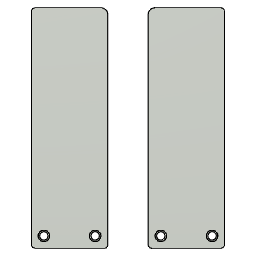
mriya-cnc-mcu-cover-v1.01 (Autodesk Fusion 360 design; units mm, degrees)
Autodesk Fusion 360 part; units mm, degrees
sketch "mriya-mcu-cover" plane through (0, 0, 0) normal (0, 0, 1) x (1, 0, 0)
  line L0 (-22.7, 5) -> (-5.8, 5) construction
  line L1 (-5, 5.8) -> (-5, 62) construction
  arc A0 (-5.8, 5) -> (-5, 5.8) centre (-5.8, 5.8) ccw construction
  arc A1 (-23.5, 5.8) -> (-22.7, 5) centre (-22.7, 5.8) ccw construction
  line L2 (-4.9, 5) -> (-4.9, 62)
  line L3 (-23.5, 5.8) -> (-23.5, 62.7) construction
  line L4 (-23.5, 63.6) -> (-6.5, 63.6)
  arc A2 (-10, 62.8) -> (-9.3, 63.5) centre (-10, 63.5) ccw construction
  arc A3 (-19.3, 63.5) -> (-18.6, 62.8) centre (-18.6, 63.5) ccw construction
  line L5 (-18.6, 62.8) -> (-10, 62.8) construction
  arc A4 (-22.7, 63.5) -> (-23.5, 62.7) centre (-22.7, 62.7) ccw construction
  line L6 (-22.7, 63.5) -> (-6.5, 63.5) construction
  line L7 (-23.5, 5) -> (-4.9, 5)
  circle A5 centre (-8, 8) radius 1.4
  circle A6 centre (-20.5, 8) radius 1.4
  line L8 (-23.5, 5) -> (-23.5, 63.6)
  arc A7 (-5, 62) -> (-6.5, 63.5) centre (-6.5, 62) ccw construction
  arc A8 (-4.9, 62) -> (-6.5, 63.6) centre (-6.5, 62) ccw
  circle A9 centre (-20.5, 8) radius 1
  circle A10 centre (-8, 8) radius 1
  line L9 (-5, 23.7) -> (-4.9, 23.7)
  dimension "d601" = 2.8
  dimension "d602" = 2.8
  dimension "d609" = 2
  dimension "d610" = 2
  constraint perpendicular L1 L6
  constraint perpendicular L0 L3
  constraint tangent A1 L3
  constraint tangent L0 A1
  constraint tangent L1 A0
  constraint tangent L0 A0
  constraint tangent L3 A4
  constraint tangent A4 L6
  constraint tangent L1 A7
  constraint tangent L6 A7
  constraint coincident L9.end L2
  constraint perpendicular L2 L7
  constraint perpendicular L4 L8
  constraint tangent A3 L5
  constraint tangent A2 L5
  constraint tangent L4 A8
  constraint tangent L2 A8
  constraint concentric A6 A9
  constraint concentric A5 A10
  constraint coincident L1 L9.start
  measures "d601" diameter of A6
  measures "d602" diameter of A5
  measures "d609" diameter of A9
  measures "d610" diameter of A10
extrude "Extrude81" add sketch "mriya-mcu-cover" along normal blind 1.5 contours L2 L4 L7 L8 A8 makes body 1
extrude "Extrude82" add sketch "mriya-mcu-cover" along normal blind 0.7 contours A5 | A6 bodies 1
fillet "Fillet60" radius 0.8 3 edges at (-23.5, 5, 0.75) (-23.5, 63.6, 0.75) (-4.9, 5, 0.75) on bodies 1
mirror "Mirror11" about plane through (0, 0, 0) normal (1, 0, 0) of bodies 1 makes body 2
named bodies: "Left", "Right"
